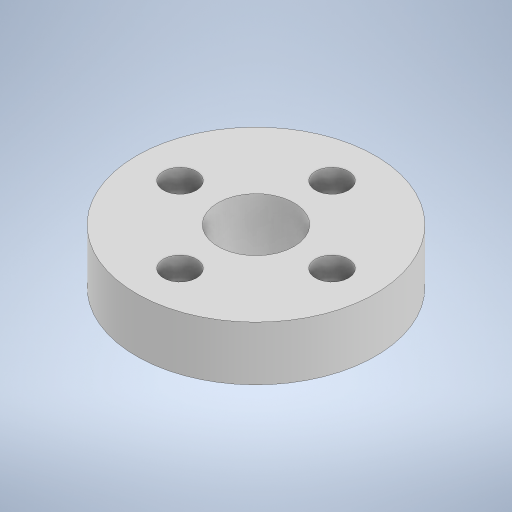
# Autodesk Inventor part: leg5
Saved by Autodesk Inventor 2024 (Build 280153000, 153)
## iProperties
Created: 2023-08-18
Part Number: leg5
Material: 常规
Document SubType Name: Modeling
Designer: wya
Density: 1 g/cm^3
Appearance: 默认
Author: wya
Autodesk Inventor part; units mm, degrees
ref_plane "YZ Plane" through (0, 0, 0) normal (1, 0, 0) x (0, 1, 0)
ref_plane "XZ Plane" through (0, 0, 0) normal (0, 1, 0) x (-1, 0, 0)
ref_plane "XY Plane" through (0, 0, 0) normal (0, 0, 1) x (1, 0, 0)
sketch "草图1" plane through (0, 0, 0) normal (0, 1, 0) x (-1, 0, 0)
  circle A0 centre (0, 0) radius 11
  circle A1 centre (0, 0) radius 7
  circle A2 centre (0, 0) radius 3.5
  circle A3 centre (7, 0) radius 1.525
  circle A4 centre (0, 7) radius 1.525
  line L0 (0, 0) -> (2.2993, 0)
  line L1 (0, 0) -> (0, -1.9489)
  circle A5 centre (0, -7) radius 1.525
  circle A6 centre (-7, 0) radius 1.525
  dimension "d0" = 22
  dimension "d1" = 14
  dimension "d2" = 7
  dimension "d3" = 3.05
  dimension "d4" = 3.05
  constraints: 7 centre point, 4 end point, 3 coincident, 2 point on circle, 2 point on line, 2 symmetric about line, 1 horizontal, 1 vertical, 2 other
  measures "d0" diameter of A0
  measures "d1" diameter of A1
  measures "d2" diameter of A2
  measures "d3" diameter of A3
  measures "d4" diameter of A4
extrude "拉伸1" add sketch "草图1" along normal blind 5 contours A0 | A3 A1 A5 A6 A4
